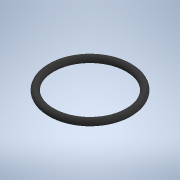
# Autodesk Inventor part: Oring 2-018 Deform
Saved by Autodesk Inventor 2020.3 (Build 243373000, 373)
## iProperties
Created: 2020-06-22
Part Number: Oring 2-018 Deform
Material: Rubber
Document SubType Name: Modeling
Designer: Bruno
Density: 0.93 g/cm^3
Appearance: Rubber - Black
Author: Bruno
Autodesk Inventor part; units mm, degrees
ref_plane "YZ Plane" through (0, 0, 0) normal (1, 0, 0) x (0, 1, 0)
ref_plane "XZ Plane" through (0, 0, 0) normal (0, 1, 0) x (-1, 0, 0)
ref_plane "XY Plane" through (0, 0, 0) normal (0, 0, 1) x (1, 0, 0)
sketch "Sketch1" plane through (0, 0, 0) normal (1, 0, 0) x (0, 1, 0)
  circle A0 centre (0, 10.39) radius 0.89
  line L0 (0, 0) -> (1.9487, 0)
  dimension "d0" = 1.78
  dimension "d1" = 10.39
  constraints: 2 end point, 1 centre point, 1 horizontal
  measures "d0" diameter of A0
  measures "d1" distance of L0.start A0.centre
revolve "Revolution1" add sketch "Sketch1" angle 360 about axis through (0, 0, 0) along (0, 1, 0)
body "Solid1"
